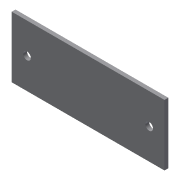
# Autodesk Inventor part: 2100-0023
Saved by Autodesk Inventor 2022 (Build 260148000, 148)
## iProperties
Shininess: 64.0
Length Units: 11269
Angle Units: 11279
Time Units: 11290
Mass Units: 11283
Length Display Precision: 3
Angle Display Precision: 2
Created: 2002-04-17
Part Number: 2100-0023
Document SubType Name: Modeling
Designer: Administrator
Density: 1 g/cm^3
Material: Generic
Appearance: Default
Density: 0.0
Volumn: 0.0
Area: 0.0
PropertySet Name: Model Information
Control State: 0
Master: False
Checked Out: False
Author: Administrator
Autodesk Inventor part; units mm, degrees
ref_plane "YZ Plane" through (0, 0, 0) normal (1, 0, 0) x (0, 1, 0)
ref_plane "XZ Plane" through (0, 0, 0) normal (0, 1, 0) x (-1, 0, 0)
ref_plane "XY Plane" through (0, 0, 0) normal (0, 0, 1) x (1, 0, 0)
sketch "Sketch1" plane through (0, 0, 0) normal (0, 0, 1) x (1, 0, 0)
  line L0 (-26.6423, 15.3027) -> (36.8577, 15.3027)
  line L1 (36.8577, 15.3027) -> (36.8577, -10.0973)
  line L2 (36.8577, -10.0973) -> (-26.6423, -10.0973)
  line L3 (-26.6423, -10.0973) -> (-26.6423, 15.3027)
  dimension "d0" = 63.5
  dimension "d1" = 25.4
  constraints: 8 end point, 2 parallel, 1 horizontal, 1 perpendicular
  measures "d0" distance of L1.end L2.end
  measures "d1" distance of L2.end L0.start
extrude "Extrusion1" add sketch "Sketch1" along normal blind 1.5875
sketch "Sketch2" plane through (0, 0, 1.5875) normal (0, 0, 1) x (1, 0, 0)
  line L0 (36.8577, 15.3027) -> (36.8577, -10.0973) projected
  line L1 (-26.6423, -10.0973) -> (-26.6423, 15.3027) projected
  line L2 (36.8577, -10.0973) -> (-26.6423, -10.0973) projected
  line L3 (-20.2923, 2.6027) -> (30.5077, 2.6027)
  circle A0 centre (5.1077, 2.6027) radius 25.4 construction
  circle A1 centre (5.1077, 2.6027) radius 31.75 construction
  dimension "d4" = 12.7
  dimension "d5" = 50.8
  constraints: 2 end point, 2 tangent, 1 centre point, 1 coincident, 1 horizontal alignment, 1 midpoint, 1 parallel, 2 other
  measures "d4" distance from line of L2 L3.start
  measures "d5" distance of L3.start L3.end
hole "Hole1" at (-20.2923, 2.6027, 1.5875) at (30.5077, 2.6027, 1.5875) direction (0, 0, -1) diameter 3.175 end through all
body "Solid1"
